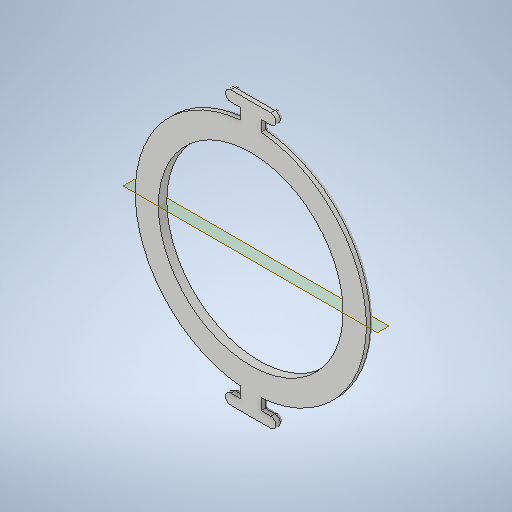
# Autodesk Inventor part: Baseplate_mitte
Saved by Autodesk Inventor 2025 (Build 290162000, 162)
## iProperties
Created: 2020-01-15
Part Number: Baseplate_mitte
Material: Generisch
Document SubType Name: Modeling
Designer: maxse
Density: 1 g/cm^3
Appearance: Vorgabe
Author: maxse
Autodesk Inventor part; units mm, degrees
(part 1 of 2)
ref_plane "YZ Plane" through (0, 0, 0) normal (1, 0, 0) x (0, 1, 0)
ref_plane "XZ Plane" through (0, 0, 0) normal (0, 1, 0) x (-1, 0, 0)
ref_plane "XY Plane" through (0, 0, 0) normal (0, 0, 1) x (1, 0, 0)
sketch "Skizze1" plane through (0, 0, 0) normal (0, 1, 0) x (-1, 0, 0)
  circle A0 centre (0, 0) radius 55
  circle A1 centre (0, 0) radius 43.96
  line L0 (-9.5, -65) -> (9.5, -65)
  line L1 (-9.5, -60) -> (-5, -60)
  line L2 (-5, -60) -> (-5, -54.7723)
  line L3 (5, -54.7723) -> (5, -60)
  line L4 (5, -60) -> (9.5, -60)
  arc A2 (9.5, -65) -> (9.5, -60) centre (9.5, -62.5) ccw
  arc A3 (-9.5, -60) -> (-9.5, -65) centre (-9.5, -62.5) ccw
  dimension "d0" = 110
  dimension "d1" = 87.92
  dimension "d2" = 10
  dimension "d3" = 2.5
  dimension "d4" = 2.5
  dimension "d5" = 5
  dimension "d6" = 5
  dimension "d7" = 24
  dimension "d8" = 60
  dimension "d9" = 4.5
  constraints: 10 end point, 6 point on circle, 4 centre point, 2 coincident, 2 horizontal, 2 point on line, 1 parallel, 1 perpendicular
  measures "d0" diameter of A0
  measures "d1" diameter of A1
  measures "d2" distance between parallel lines of L3 L2
  measures "d3" radius of A2
  measures "d4" radius of A3
  measures "d5" distance between parallel lines of L1 L0
  measures "d6" distance from line of point (0, 0) L2
  measures "d8" distance from line of A0.centre L4
  measures "d9" distance from line of L3 A2.centre
extrude "Extrusion1" add sketch "Skizze1" along normal blind 4
mirror "Spiegeln1" about plane through (0, 0, 0) normal (0, 0, 1) of "Extrusion1"
fillet "Rundung2" radius 2 16 edges at (-55, 4, 0) (55, 4, 0) (5, 4, 57.3861) (-5, 4, 57.3861) (-12, 4, 62.5) (-7.25, 4, 60) (12, 4, 62.5) (7.25, 4, 60) (0, 4, 65) (-12, 4, -62.5) (-7.25, 4, -60) (12, 4, -62.5) (7.25, 4, -60) (0, 4, -65) (-5, 4, -57.3861) (5, 4, -57.3861)
sketch "Skizze2" plane through (0, 4, 0) normal (0, 1, 0) x (1, 0, 0)
  circle A0 centre (0, 0) radius 45 projected
  line L0 (-69.5668, 0) -> (60.0552, 0)
  spline S0 degree 2 poles (24.3984, -40.0383) (24.7167, -39.8443) (25.3552, -39.7162) (25.6461, -39.781) knots 0 0 0 1 2 2 2
  spline S1 degree 2 poles (25.6461, -39.781) (25.9314, -39.8443) (26.405, -40.201) (26.5674, -40.4675) knots 0 0 0 1 2 2 2
  spline S2 degree 2 poles (26.5674, -40.4675) (26.7782, -40.8135) (26.7622, -41.6204) (26.5147, -42.0084) knots 0 0 0 1 2 2 2
  line L1 (26.5147, -42.0084) -> (26.5253, -42.0257)
  spline S3 degree 2 poles (26.5253, -42.0257) (26.9519, -42.0172) (27.522, -42.2677) (27.7202, -42.5929) knots 0 0 0 1 2 2 2
  spline S4 degree 2 poles (27.7202, -42.5929) (28.0133, -43.0738) (27.6789, -44.1602) (27.1183, -44.5018) knots 0 0 0 1 2 2 2
  spline S5 degree 2 poles (27.1183, -44.5018) (26.5371, -44.856) (25.4636, -44.675) (25.1726, -44.1976) knots 0 0 0 1 2 2 2
  spline S6 degree 2 poles (25.1726, -44.1976) (24.9976, -43.9104) (24.9917, -43.1453) (25.2095, -42.7943) knots 0 0 0 1 2 2 2
  line L2 (25.2095, -42.7943) -> (25.199, -42.777)
  spline S7 degree 2 poles (25.199, -42.777) (24.7199, -42.8317) (24.0322, -42.5675) (23.7918, -42.173) knots 0 0 0 1 2 2 2
  spline S8 degree 2 poles (23.7918, -42.173) (23.4587, -41.6264) (23.8033, -40.401) (24.3984, -40.0383) knots 0 0 0 1 2 2 2
  spline S9 degree 2 poles (24.3463, -41.7592) (24.5065, -42.0222) (24.9039, -42.2071) (25.295, -42.187) knots 0 0 0 1 2 2 2
  spline S10 degree 2 poles (25.295, -42.187) (25.4256, -42.1834) (25.8289, -42.1132) (26.0836, -42.0718) knots 0 0 0 1 2 2 2
  spline S11 degree 2 poles (26.0836, -42.0718) (26.224, -41.7728) (26.1941, -41.1552) (26.0149, -40.8611) knots 0 0 0 1 2 2 2
  spline S12 degree 2 poles (26.0149, -40.8611) (25.7787, -40.4736) (25.0038, -40.253) (24.6508, -40.4681) knots 0 0 0 1 2 2 2
  spline S13 degree 2 poles (24.6508, -40.4681) (24.291, -40.6874) (24.1186, -41.3856) (24.3463, -41.7592) knots 0 0 0 1 2 2 2
  spline S14 degree 2 poles (25.7289, -43.8491) (25.9039, -44.1362) (26.522, -44.2863) (26.8646, -44.0775) knots 0 0 0 1 2 2 2
  spline S15 degree 2 poles (26.8646, -44.0775) (27.176, -43.8878) (27.3651, -43.3028) (27.1859, -43.0086) knots 0 0 0 1 2 2 2
  spline S16 degree 2 poles (27.1859, -43.0086) (27.0573, -42.7976) (26.6739, -42.6279) (26.3981, -42.6346) knots 0 0 0 1 2 2 2
  spline S17 degree 2 poles (26.3981, -42.6346) (26.2821, -42.6389) (25.812, -42.6929) (25.6337, -42.7351) knots 0 0 0 1 2 2 2
  spline S18 degree 2 poles (25.6337, -42.7351) (25.5006, -43.0772) (25.5708, -43.5896) (25.7289, -43.8491) knots 0 0 0 1 2 2 2
  line L3 (21.6421, -46.4852) -> (21.6582, -41.7158)
  line L4 (21.6582, -41.7158) -> (22.2948, -41.3944)
  line L5 (22.2948, -41.3944) -> (22.2433, -46.3633)
  line L6 (22.2433, -46.3633) -> (24.5473, -45.2002)
  line L7 (24.5473, -45.2002) -> (24.8121, -45.7246)
  line L8 (24.8121, -45.7246) -> (21.9799, -47.1544)
  line L9 (21.9799, -47.1544) -> (21.6421, -46.4852)
  line L10 (18.1735, -43.3461) -> (18.9107, -43.0296)
  line L11 (18.9107, -43.0296) -> (19.2879, -43.9083)
  line L12 (19.2879, -43.9083) -> (18.5507, -44.2248)
  line L13 (18.5507, -44.2248) -> (18.1735, -43.3461)
  spline S19 degree 2 poles (14.9287, -46.263) (14.8073, -45.9235) (14.8174, -45.2658) (14.9394, -44.9812) knots 0 0 0 1 2 2 2
  spline S20 degree 2 poles (14.9394, -44.9812) (15.0614, -44.6966) (15.5641, -44.2371) (15.9304, -44.1062) knots 0 0 0 1 2 2 2
  spline S21 degree 2 poles (15.9304, -44.1062) (16.2661, -43.9861) (16.9756, -43.9003) (17.2582, -43.9326) knots 0 0 0 1 2 2 2
  line L14 (17.2582, -43.9326) -> (17.497, -44.6003)
  line L15 (17.497, -44.6003) -> (17.4512, -44.6166)
  spline S22 degree 2 poles (17.4512, -44.6166) (17.3596, -44.5891) (17.0396, -44.5487) (16.8537, -44.5463) knots 0 0 0 1 2 2 2
  spline S23 degree 2 poles (16.8537, -44.5463) (16.6436, -44.5483) (16.3086, -44.5863) (16.114, -44.6558) knots 0 0 0 1 2 2 2
  spline S24 degree 2 poles (16.114, -44.6558) (15.9233, -44.7241) (15.6137, -44.9896) (15.5372, -45.1848) knots 0 0 0 1 2 2 2
  spline S25 degree 2 poles (15.5372, -45.1848) (15.4694, -45.3683) (15.481, -45.7858) (15.5711, -46.0376) knots 0 0 0 1 2 2 2
  spline S26 degree 2 poles (15.5711, -46.0376) (15.6611, -46.2895) (15.9131, -46.5608) (16.081, -46.6213) knots 0 0 0 1 2 2 2
  spline S27 degree 2 poles (16.081, -46.6213) (16.2568, -46.6918) (16.6891, -46.6491) (16.9294, -46.5632) knots 0 0 0 1 2 2 2
  spline S28 degree 2 poles (16.9294, -46.5632) (17.1889, -46.4704) (17.6753, -46.2061) (17.8194, -46.1158) knots 0 0 0 1 2 2 2
  line L16 (17.8194, -46.1158) -> (18.6871, -48.5424)
  line L17 (18.6871, -48.5424) -> (16.1041, -49.466)
  line L18 (16.1041, -49.466) -> (15.9063, -48.9127)
  line L19 (15.9063, -48.9127) -> (17.8826, -48.2061)
  line L20 (17.8826, -48.2061) -> (17.4338, -46.9508)
  spline S29 degree 2 poles (17.4338, -46.9508) (17.3248, -47.007) (17.1076, -47.0976) (17.016, -47.1303) knots 0 0 0 1 2 2 2
  spline S30 degree 2 poles (17.016, -47.1303) (16.6536, -47.2599) (16.1115, -47.3204) (15.8198, -47.2267) knots 0 0 0 1 2 2 2
  spline S31 degree 2 poles (15.8198, -47.2267) (15.5243, -47.1344) (15.0815, -46.6903) (14.9287, -46.263) knots 0 0 0 1 2 2 2
  line L21 (9.4987, -46.0663) -> (10.0195, -48.1748)
  spline S32 degree 2 poles (10.0195, -48.1748) (10.0817, -48.4265) (10.2269, -48.8456) (10.319, -48.948) knots 0 0 0 1 2 2 2
  spline S33 degree 2 poles (10.319, -48.948) (10.414, -49.0623) (10.685, -49.1289) (10.8935, -49.0774) knots 0 0 0 1 2 2 2
  spline S34 degree 2 poles (10.8935, -49.0774) (11.0823, -49.0308) (11.4577, -48.6918) (11.6315, -48.4152) knots 0 0 0 1 2 2 2
  spline S35 degree 2 poles (11.6315, -48.4152) (11.6139, -48.3611) (11.5682, -48.2096) (11.5429, -48.1073) knots 0 0 0 1 2 2 2
  line L22 (11.5429, -48.1073) -> (10.9502, -45.7078)
  line L23 (10.9502, -45.7078) -> (11.5638, -45.5562)
  line L24 (11.5638, -45.5562) -> (12.0846, -47.6646)
  spline S36 degree 2 poles (12.0846, -47.6646) (12.1468, -47.9164) (12.2921, -48.3354) (12.3842, -48.4379) knots 0 0 0 1 2 2 2
  spline S37 degree 2 poles (12.3842, -48.4379) (12.4792, -48.5522) (12.7502, -48.6188) (12.9587, -48.5673) knots 0 0 0 1 2 2 2
  spline S38 degree 2 poles (12.9587, -48.5673) (13.1554, -48.5187) (13.5308, -48.163) (13.6877, -47.9198) knots 0 0 0 1 2 2 2
  line L25 (13.6877, -47.9198) -> (13.0153, -45.1977)
  line L26 (13.0153, -45.1977) -> (13.629, -45.0461)
  line L27 (13.629, -45.0461) -> (14.5287, -48.6886)
  line L28 (14.5287, -48.6886) -> (13.9151, -48.8402)
  line L29 (13.9151, -48.8402) -> (13.816, -48.439)
  spline S39 degree 2 poles (13.816, -48.439) (13.6353, -48.7382) (13.2284, -49.1184) (12.9451, -49.1883) knots 0 0 0 1 2 2 2
  spline S40 degree 2 poles (12.9451, -49.1883) (12.6226, -49.268) (12.0501, -49.0964) (11.8377, -48.7941) knots 0 0 0 1 2 2 2
  spline S41 degree 2 poles (11.8377, -48.7941) (11.6352, -49.1738) (11.1868, -49.6227) (10.88, -49.6984) knots 0 0 0 1 2 2 2
  spline S42 degree 2 poles (10.88, -49.6984) (10.644, -49.7567) (10.2225, -49.7064) (10.0401, -49.5762) knots 0 0 0 1 2 2 2
  spline S43 degree 2 poles (10.0401, -49.5762) (9.8537, -49.4469) (9.57, -48.9911) (9.4777, -48.6174) knots 0 0 0 1 2 2 2
  line L30 (9.4777, -48.6174) -> (8.885, -46.2179)
  line L31 (8.885, -46.2179) -> (9.4987, -46.0663)
  line L32 (3.7893, -46.8825) -> (4.0482, -49.0389)
  spline S44 degree 2 poles (4.0482, -49.0389) (4.0791, -49.2963) (4.172, -49.73) (4.2508, -49.843) knots 0 0 0 1 2 2 2
  spline S45 degree 2 poles (4.2508, -49.843) (4.3311, -49.968) (4.592, -50.0673) (4.8052, -50.0417) knots 0 0 0 1 2 2 2
  spline S46 degree 2 poles (4.8052, -50.0417) (4.9983, -50.0185) (5.4123, -49.728) (5.6186, -49.4747) knots 0 0 0 1 2 2 2
  spline S47 degree 2 poles (5.6186, -49.4747) (5.6078, -49.4189) (5.5809, -49.263) (5.5684, -49.1584) knots 0 0 0 1 2 2 2
  line L33 (5.5684, -49.1584) -> (5.2738, -46.7043)
  line L34 (5.2738, -46.7043) -> (5.9014, -46.629)
  line L35 (5.9014, -46.629) -> (6.1602, -48.7853)
  spline S48 degree 2 poles (6.1602, -48.7853) (6.1911, -49.0428) (6.284, -49.4765) (6.3629, -49.5894) knots 0 0 0 1 2 2 2
  spline S49 degree 2 poles (6.3629, -49.5894) (6.4432, -49.7145) (6.704, -49.8137) (6.9172, -49.7882) knots 0 0 0 1 2 2 2
  spline S50 degree 2 poles (6.9172, -49.7882) (7.1184, -49.764) (7.5345, -49.457) (7.7201, -49.2347) knots 0 0 0 1 2 2 2
  line L36 (7.7201, -49.2347) -> (7.3859, -46.4508)
  line L37 (7.3859, -46.4508) -> (8.0135, -46.3755)
  line L38 (8.0135, -46.3755) -> (8.4606, -50.1008)
  line L39 (8.4606, -50.1008) -> (7.8331, -50.1761)
  line L40 (7.8331, -50.1761) -> (7.7838, -49.7658)
  spline S51 degree 2 poles (7.7838, -49.7658) (7.5679, -50.0406) (7.1175, -50.3681) (6.8278, -50.4029) knots 0 0 0 1 2 2 2
  spline S52 degree 2 poles (6.8278, -50.4029) (6.4979, -50.4425) (5.9508, -50.2021) (5.777, -49.8761) knots 0 0 0 1 2 2 2
  spline S53 degree 2 poles (5.777, -49.8761) (5.5295, -50.2282) (5.0295, -50.6187) (4.7157, -50.6564) knots 0 0 0 1 2 2 2
  spline S54 degree 2 poles (4.7157, -50.6564) (4.4744, -50.6854) (4.0622, -50.5839) (3.8971, -50.4323) knots 0 0 0 1 2 2 2
  spline S55 degree 2 poles (3.8971, -50.4323) (3.728, -50.2812) (3.5022, -49.7941) (3.4563, -49.4119) knots 0 0 0 1 2 2 2
  line L41 (3.4563, -49.4119) -> (3.1617, -46.9579)
  line L42 (3.1617, -46.9579) -> (3.7893, -46.8825)
  spline S56 degree 2 poles (-3.071, -48.9106) (-3.0447, -47.9709) (-2.1185, -46.8862) (-1.434, -46.9053) knots 0 0 0 1 2 2 2
  spline S57 degree 2 poles (-1.434, -46.9053) (-1.1545, -46.9131) (-0.7288, -47.0547) (-0.5098, -47.1946) knots 0 0 0 1 2 2 2
  line L43 (-0.5098, -47.1946) -> (-0.4658, -45.6231)
  line L44 (-0.4658, -45.6231) -> (0.166, -45.6408)
  line L45 (0.166, -45.6408) -> (0.0224, -50.7725)
  line L46 (0.0224, -50.7725) -> (-0.6094, -50.7548)
  line L47 (-0.6094, -50.7548) -> (-0.5984, -50.362)
  spline S58 degree 2 poles (-0.5984, -50.362) (-0.8393, -50.5701) (-1.4224, -50.8375) (-1.7586, -50.8281) knots 0 0 0 1 2 2 2
  spline S59 degree 2 poles (-1.7586, -50.8281) (-2.4026, -50.8101) (-3.095, -49.7692) (-3.071, -48.9106) knots 0 0 0 1 2 2 2
  spline S60 degree 2 poles (-2.4168, -48.8559) (-2.4348, -49.4999) (-2.0456, -50.2201) (-1.5879, -50.2329) knots 0 0 0 1 2 2 2
  spline S61 degree 2 poles (-1.5879, -50.2329) (-1.3206, -50.2404) (-0.8117, -50.0155) (-0.5837, -49.8354) knots 0 0 0 1 2 2 2
  line L48 (-0.5837, -49.8354) -> (-0.5241, -47.705)
  spline S62 degree 2 poles (-0.5241, -47.705) (-0.7679, -47.5806) (-1.1177, -47.4816) (-1.3446, -47.4753) knots 0 0 0 1 2 2 2
  spline S63 degree 2 poles (-1.3446, -47.4753) (-1.8346, -47.4616) (-2.3976, -48.1673) (-2.4168, -48.8559) knots 0 0 0 1 2 2 2
  spline S64 degree 2 poles (-5.2796, -46.6177) (-4.3852, -46.7137) (-3.5098, -47.8223) (-3.6092, -48.7489) knots 0 0 0 1 2 2 2
  spline S65 degree 2 poles (-3.6092, -48.7489) (-3.7069, -49.6594) (-4.7775, -50.6367) (-5.547, -50.5541) knots 0 0 0 1 2 2 2
  spline S66 degree 2 poles (-5.547, -50.5541) (-5.8935, -50.517) (-6.4077, -50.258) (-6.5822, -50.0233) knots 0 0 0 1 2 2 2
  spline S67 degree 2 poles (-6.5822, -50.0233) (-6.7607, -49.7882) (-6.9081, -49.1489) (-6.8601, -48.7017) knots 0 0 0 1 2 2 2
  line L49 (-6.8601, -48.7017) -> (-6.8234, -48.3593)
  line L50 (-6.8234, -48.3593) -> (-4.241, -48.6363)
  spline S68 degree 2 poles (-4.241, -48.6363) (-4.1714, -47.9876) (-4.7502, -47.2287) (-5.3303, -47.1665) knots 0 0 0 1 2 2 2
  spline S69 degree 2 poles (-5.3303, -47.1665) (-5.5358, -47.1445) (-5.9446, -47.1943) (-6.1135, -47.2496) knots 0 0 0 1 2 2 2
  spline S70 degree 2 poles (-6.1135, -47.2496) (-6.2913, -47.312) (-6.5401, -47.4279) (-6.6236, -47.4842) knots 0 0 0 1 2 2 2
  line L51 (-6.6236, -47.4842) -> (-6.6599, -47.4803)
  line L52 (-6.6599, -47.4803) -> (-6.5864, -46.7954)
  spline S71 degree 2 poles (-6.5864, -46.7954) (-6.4729, -46.7628) (-6.1287, -46.6693) (-5.9959, -46.6468) knots 0 0 0 1 2 2 2
  spline S72 degree 2 poles (-5.9959, -46.6468) (-5.809, -46.6139) (-5.5052, -46.5935) (-5.2796, -46.6177) knots 0 0 0 1 2 2 2
  spline S73 degree 2 poles (-6.2625, -48.9044) (-6.2816, -49.1591) (-6.2166, -49.5409) (-6.1293, -49.6766) knots 0 0 0 1 2 2 2
  spline S74 degree 2 poles (-6.1293, -49.6766) (-6.0357, -49.8293) (-5.7092, -50.0151) (-5.4554, -50.0423) knots 0 0 0 1 2 2 2
  spline S75 degree 2 poles (-5.4554, -50.0423) (-5.2056, -50.0691) (-4.8391, -49.9577) (-4.6785, -49.8282) knots 0 0 0 1 2 2 2
  spline S76 degree 2 poles (-4.6785, -49.8282) (-4.5215, -49.6942) (-4.3381, -49.3512) (-4.2924, -49.1157) knots 0 0 0 1 2 2 2
  line L53 (-4.2924, -49.1157) -> (-6.2625, -48.9044)
  spline S77 degree 2 poles (-8.3657, -46.1775) (-7.8585, -46.2644) (-7.3867, -46.9414) (-7.4942, -47.5684) knots 0 0 0 1 2 2 2
  line L54 (-7.4942, -47.5684) -> (-7.8455, -49.6171)
  line L55 (-7.8455, -49.6171) -> (-7.4262, -49.689)
  line L56 (-7.4262, -49.689) -> (-7.5145, -50.2042)
  line L57 (-7.5145, -50.2042) -> (-7.9338, -50.1323)
  line L58 (-7.9338, -50.1323) -> (-8.116, -51.1946)
  line L59 (-8.116, -51.1946) -> (-8.739, -51.0878)
  line L60 (-8.739, -51.0878) -> (-8.5568, -50.0255)
  line L61 (-8.5568, -50.0255) -> (-9.703, -49.829)
  line L62 (-9.703, -49.829) -> (-9.6146, -49.3138)
  line L63 (-9.6146, -49.3138) -> (-8.4685, -49.5103)
  line L64 (-8.4685, -49.5103) -> (-8.1665, -47.7491)
  spline S78 degree 2 poles (-8.1665, -47.7491) (-8.1186, -47.4696) (-8.0858, -47.1587) (-8.1311, -47.0152) knots 0 0 0 1 2 2 2
  spline S79 degree 2 poles (-8.1311, -47.0152) (-8.1672, -46.8898) (-8.3989, -46.7309) (-8.6146, -46.6939) knots 0 0 0 1 2 2 2
  spline S80 degree 2 poles (-8.6146, -46.6939) (-8.7663, -46.6679) (-9.0656, -46.7111) (-9.1343, -46.7281) knots 0 0 0 1 2 2 2
  line L65 (-9.1343, -46.7281) -> (-9.1703, -46.722)
  line L66 (-9.1703, -46.722) -> (-9.0744, -46.1629)
  spline S81 degree 2 poles (-9.0744, -46.1629) (-8.8905, -46.1451) (-8.5214, -46.1508) (-8.3657, -46.1775) knots 0 0 0 1 2 2 2
  line L67 (-12.1384, -48.5969) -> (-12.1068, -48.604)
  spline S82 degree 2 poles (-12.1068, -48.604) (-12.0401, -48.6397) (-11.8877, -48.6822) (-11.7809, -48.7062) knots 0 0 0 1 2 2 2
  spline S83 degree 2 poles (-11.7809, -48.7062) (-11.5318, -48.762) (-10.9928, -48.6546) (-10.7235, -48.4907) knots 0 0 0 1 2 2 2
  line L68 (-10.7235, -48.4907) -> (-10.1409, -45.8932)
  line L69 (-10.1409, -45.8932) -> (-9.5241, -46.0315)
  line L70 (-9.5241, -46.0315) -> (-10.3453, -49.6926)
  line L71 (-10.3453, -49.6926) -> (-10.9621, -49.5542)
  line L72 (-10.9621, -49.5542) -> (-10.8397, -49.0086)
  spline S84 degree 2 poles (-10.8397, -49.0086) (-11.2432, -49.2337) (-11.8003, -49.3662) (-12.0375, -49.313) knots 0 0 0 1 2 2 2
  spline S85 degree 2 poles (-12.0375, -49.313) (-12.1324, -49.2917) (-12.2255, -49.2625) (-12.2821, -49.2374) knots 0 0 0 1 2 2 2
  line L73 (-12.2821, -49.2374) -> (-12.1384, -48.5969)
  line L74 (-12.5586, -45.2922) -> (-11.9483, -45.457)
  line L75 (-11.9483, -45.457) -> (-12.9265, -49.0793)
  line L76 (-12.9265, -49.0793) -> (-13.5367, -48.9145)
  line L77 (-13.5367, -48.9145) -> (-12.5586, -45.2922)
  line L78 (-13.7425, -49.5052) -> (-13.0501, -49.6922)
  line L79 (-13.0501, -49.6922) -> (-13.2212, -50.3259)
  line L80 (-13.2212, -50.3259) -> (-13.9136, -50.1389)
  line L81 (-13.9136, -50.1389) -> (-13.7425, -49.5052)
  line L82 (-18.1924, -43.3603) -> (-17.6023, -43.5869)
  line L83 (-17.6023, -43.5869) -> (-17.7388, -43.9424)
  spline S86 degree 2 poles (-17.7388, -43.9424) (-17.5591, -43.8812) (-17.3005, -43.8069) (-17.1396, -43.7949) knots 0 0 0 1 2 2 2
  spline S87 degree 2 poles (-17.1396, -43.7949) (-16.9916, -43.7823) (-16.6983, -43.8211) (-16.5205, -43.8893) knots 0 0 0 1 2 2 2
  spline S88 degree 2 poles (-16.5205, -43.8893) (-16.2331, -43.9997) (-15.8404, -44.4239) (-15.7587, -44.72) knots 0 0 0 1 2 2 2
  spline S89 degree 2 poles (-15.7587, -44.72) (-15.6771, -45.0161) (-15.7494, -45.7696) (-15.9193, -46.2122) knots 0 0 0 1 2 2 2
  spline S90 degree 2 poles (-15.9193, -46.2122) (-16.0965, -46.6737) (-16.5933, -47.2555) (-16.8986, -47.429) knots 0 0 0 1 2 2 2
  spline S91 degree 2 poles (-16.8986, -47.429) (-17.1787, -47.5819) (-17.8198, -47.6353) (-18.1186, -47.5205) knots 0 0 0 1 2 2 2
  spline S92 degree 2 poles (-18.1186, -47.5205) (-18.3797, -47.4203) (-18.7242, -47.1535) (-18.8934, -46.9497) knots 0 0 0 1 2 2 2
  line L84 (-18.8934, -46.9497) -> (-19.4743, -48.4627)
  line L85 (-19.4743, -48.4627) -> (-20.0644, -48.2362)
  line L86 (-20.0644, -48.2362) -> (-18.1924, -43.3603)
  line L87 (-17.9291, -44.438) -> (-18.706, -46.4617)
  spline S93 degree 2 poles (-18.706, -46.4617) (-18.5273, -46.6518) (-18.2098, -46.8649) (-18.0093, -46.9419) knots 0 0 0 1 2 2 2
  spline S94 degree 2 poles (-18.0093, -46.9419) (-17.5554, -47.1161) (-16.7796, -46.6328) (-16.5327, -45.9897) knots 0 0 0 1 2 2 2
  spline S95 degree 2 poles (-16.5327, -45.9897) (-16.2945, -45.3693) (-16.4366, -44.5639) (-16.8717, -44.3969) knots 0 0 0 1 2 2 2
  spline S96 degree 2 poles (-16.8717, -44.3969) (-17.1024, -44.3083) (-17.6528, -44.3401) (-17.9291, -44.438) knots 0 0 0 1 2 2 2
  line L88 (-19.6119, -42.7139) -> (-19.0357, -42.9737)
  line L89 (-19.0357, -42.9737) -> (-20.5783, -46.394)
  line L90 (-20.5783, -46.394) -> (-21.1545, -46.1341)
  line L91 (-21.1545, -46.1341) -> (-19.6119, -42.7139)
  line L92 (-21.4517, -46.6846) -> (-20.7979, -46.9794)
  line L93 (-20.7979, -46.9794) -> (-21.0678, -47.5778)
  line L94 (-21.0678, -47.5778) -> (-21.7216, -47.2829)
  line L95 (-21.7216, -47.2829) -> (-21.4517, -46.6846)
  spline S97 degree 2 poles (-21.3169, -41.7878) (-20.9815, -41.9595) (-20.4931, -42.4371) (-20.3536, -42.6359) knots 0 0 0 1 2 2 2
  line L96 (-20.3536, -42.6359) -> (-20.6766, -43.2671)
  line L97 (-20.6766, -43.2671) -> (-20.7055, -43.2523)
  spline S98 degree 2 poles (-20.7055, -43.2523) (-20.7481, -43.1577) (-20.8727, -42.921) (-20.9963, -42.7621) knots 0 0 0 1 2 2 2
  spline S99 degree 2 poles (-20.9963, -42.7621) (-21.1019, -42.6216) (-21.3964, -42.3434) (-21.5804, -42.2493) knots 0 0 0 1 2 2 2
  spline S100 degree 2 poles (-21.5804, -42.2493) (-21.7138, -42.1809) (-22.0518, -42.0854) (-22.1498, -42.0989) knots 0 0 0 1 2 2 2
  spline S101 degree 2 poles (-22.1498, -42.0989) (-22.2895, -42.1139) (-22.4626, -42.221) (-22.5438, -42.3797) knots 0 0 0 1 2 2 2
  spline S102 degree 2 poles (-22.5438, -42.3797) (-22.6454, -42.5781) (-22.5342, -42.8945) (-22.2915, -43.1051) knots 0 0 0 1 2 2 2
  spline S103 degree 2 poles (-22.2915, -43.1051) (-22.1962, -43.1858) (-21.8869, -43.4351) (-21.7593, -43.5505) knots 0 0 0 1 2 2 2
  spline S104 degree 2 poles (-21.7593, -43.5505) (-21.4342, -43.858) (-21.3243, -44.4969) (-21.4922, -44.8251) knots 0 0 0 1 2 2 2
  spline S105 degree 2 poles (-21.4922, -44.8251) (-21.7249, -45.2796) (-22.6964, -45.497) (-23.2591, -45.209) knots 0 0 0 1 2 2 2
  spline S106 degree 2 poles (-23.2591, -45.209) (-23.5368, -45.0668) (-24.0293, -44.6418) (-24.1669, -44.4393) knots 0 0 0 1 2 2 2
  line L98 (-24.1669, -44.4393) -> (-23.8587, -43.837)
  line L99 (-23.8587, -43.837) -> (-23.8298, -43.8518)
  spline S107 degree 2 poles (-23.8298, -43.8518) (-23.702, -44.1357) (-23.2769, -44.6036) (-23.0064, -44.742) knots 0 0 0 1 2 2 2
  spline S108 degree 2 poles (-23.0064, -44.742) (-22.7287, -44.8842) (-22.2264, -44.8454) (-22.1064, -44.6109) knots 0 0 0 1 2 2 2
  spline S109 degree 2 poles (-22.1064, -44.6109) (-21.9974, -44.3981) (-22.1195, -44.0762) (-22.3387, -43.8821) knots 0 0 0 1 2 2 2
  spline S110 degree 2 poles (-22.3387, -43.8821) (-22.4447, -43.7869) (-22.7217, -43.5632) (-22.8709, -43.4367) knots 0 0 0 1 2 2 2
  spline S111 degree 2 poles (-22.8709, -43.4367) (-23.1908, -43.1547) (-23.3463, -42.5335) (-23.1561, -42.1619) knots 0 0 0 1 2 2 2
  spline S112 degree 2 poles (-23.1561, -42.1619) (-23.0453, -41.9455) (-22.6801, -41.65) (-22.4422, -41.5942) knots 0 0 0 1 2 2 2
  spline S113 degree 2 poles (-22.4422, -41.5942) (-22.1898, -41.5368) (-21.6596, -41.6124) (-21.3169, -41.7878) knots 0 0 0 1 2 2 2
  line L100 (-25.6934, -39.3835) -> (-25.1534, -39.712)
  line L101 (-25.1534, -39.712) -> (-26.2651, -41.5398)
  spline S114 degree 2 poles (-26.2651, -41.5398) (-26.3998, -41.7614) (-26.5899, -42.1675) (-26.597, -42.3196) knots 0 0 0 1 2 2 2
  spline S115 degree 2 poles (-26.597, -42.3196) (-26.605, -42.4808) (-26.4411, -42.7416) (-26.2403, -42.8638) knots 0 0 0 1 2 2 2
  spline S116 degree 2 poles (-26.2403, -42.8638) (-26.0396, -42.9859) (-25.4832, -43.0302) (-25.1737, -42.9814) knots 0 0 0 1 2 2 2
  line L102 (-25.1737, -42.9814) -> (-23.7167, -40.5857)
  line L103 (-23.7167, -40.5857) -> (-23.1766, -40.9142)
  line L104 (-23.1766, -40.9142) -> (-25.8906, -45.3765)
  line L105 (-25.8906, -45.3765) -> (-26.4307, -45.0481)
  line L106 (-26.4307, -45.0481) -> (-25.4495, -43.4349)
  spline S117 degree 2 poles (-25.4495, -43.4349) (-25.8245, -43.5056) (-26.4308, -43.4498) (-26.6939, -43.2898) knots 0 0 0 1 2 2 2
  spline S118 degree 2 poles (-26.6939, -43.2898) (-27.1647, -43.0034) (-27.3188, -42.0561) (-26.9588, -41.4641) knots 0 0 0 1 2 2 2
  line L107 (-26.9588, -41.4641) -> (-25.6934, -39.3835)
  point P0 (0, 0)
  constraints: 2 end point, 1 horizontal, 2 other
extrude "Extrusion2" add sketch "Skizze2" along normal blind 1 contours S0 S1 S2 L1 S3 S4 S5 S6 L2 S7 S8 | L3 L4 L5 L6 L7 L8 L9 | L10 L11 L12 L13 | S19 S20 S21 L14 L15 S22 S23 S24 S25 S26 S27 S28 L16 L17 L18 L19 L20 S29 S30 S31 | L21 S32 S33 S34 S35 L22 L23 L24 S36 S37 S38 L25 L26 L27 L28 L29 S39 S40 S41 S42 S43 L30 L31 | L32 S44 S45 S46 S47 L33 L34 L35 S48 S49 S50 L36 L37 L38 L39 L40 S51 S52 S53 S54 S55 L41 L42 | S56 S57 L43 L44 L45 L46 L47 S58 S59 | S64 S65 S66 S67 L49 L50 S68 S69 S70 L51 L52 S71 S72 | S77 L54 L55 L56 L57 L58 L59 L60 L61 L62 L63 L64 S78 S79 S80 L65 L66 S81 | L67 S82 S83 L68 L69 L70 L71 L72 S84 S85 L73 | L74 L75 L76 L77 | L78 L79 L80 L81 | L82 L83 S86 S87 S88 S89 S90 S91 S92 L84 L85 L86 | L88 L89 L90 L91 | L92 L93 L94 L95 | S97 L96 L97 S98 S99 S100 S101 S102 S103 S104 S105 S106 L98 L99 S107 S108 S109 S110 S111 S112 S113 | L100 L101 S114 S115 S116 L102 L103 L104 L105 L106 S117 S118 L107
sketch "Skizze3" plane through (0, 4, 0) normal (0, 1, 0) x (1, 0, 0)
  circle A0 centre (0, 0) radius 45.2717
  spline S0 degree 2 poles (28.1118, 38.7127) (28.2498, 38.8928) (28.6266, 39.1186) (28.8277, 39.1431) knots 0 0 0 1 2 2 2
  spline S1 degree 2 poles (28.8277, 39.1431) (29.0804, 39.1745) (29.582, 39.0223) (29.8792, 38.7946) knots 0 0 0 1 2 2 2
  line L0 (29.8792, 38.7946) -> (30.1921, 38.5547)
  line L1 (30.1921, 38.5547) -> (30.9858, 39.5902)
  line L2 (30.9858, 39.5902) -> (31.355, 39.3072)
  line L3 (31.355, 39.3072) -> (29.2257, 36.5294)
  line L4 (29.2257, 36.5294) -> (28.5279, 37.0643)
  spline S2 degree 2 poles (28.5279, 37.0643) (28.2803, 37.2541) (27.9957, 37.6009) (27.9337, 37.795) knots 0 0 0 1 2 2 2
  spline S3 degree 2 poles (27.9337, 37.795) (27.8594, 38.0198) (27.934, 38.4808) (28.1118, 38.7127) knots 0 0 0 1 2 2 2
  spline S4 degree 2 poles (28.5053, 38.4289) (28.3949, 38.2848) (28.3318, 37.9973) (28.3813, 37.8521) knots 0 0 0 1 2 2 2
  spline S5 degree 2 poles (28.3813, 37.8521) (28.4242, 37.7263) (28.6221, 37.4996) (28.7954, 37.3667) knots 0 0 0 1 2 2 2
  line L5 (28.7954, 37.3667) -> (29.1016, 37.132)
  line L6 (29.1016, 37.132) -> (29.9505, 38.2396)
  line L7 (29.9505, 38.2396) -> (29.6984, 38.4328)
  spline S6 degree 2 poles (29.6984, 38.4328) (29.4733, 38.6054) (29.1412, 38.7456) (28.9787, 38.72) knots 0 0 0 1 2 2 2
  spline S7 degree 2 poles (28.9787, 38.72) (28.8315, 38.7006) (28.6071, 38.5617) (28.5053, 38.4289) knots 0 0 0 1 2 2 2
  spline S8 degree 2 poles (27.9009, 41.4872) (27.9678, 41.4894) (28.1977, 41.5034) (28.292, 41.4902) knots 0 0 0 1 2 2 2
  spline S9 degree 2 poles (28.292, 41.4902) (28.4231, 41.4757) (28.64, 41.4057) (28.8036, 41.2932) knots 0 0 0 1 2 2 2
  spline S10 degree 2 poles (28.8036, 41.2932) (28.9368, 41.2016) (29.1084, 40.9356) (29.1369, 40.7817) knots 0 0 0 1 2 2 2
  spline S11 degree 2 poles (29.1369, 40.7817) (29.1623, 40.6335) (29.0874, 40.2994) (28.9878, 40.1545) knots 0 0 0 1 2 2 2
  spline S12 degree 2 poles (28.9878, 40.1545) (28.8335, 39.9302) (28.4256, 39.7425) (28.1573, 39.7928) knots 0 0 0 1 2 2 2
  spline S13 degree 2 poles (28.1573, 39.7928) (27.9171, 39.834) (27.3783, 40.1117) (27.0796, 40.293) knots 0 0 0 1 2 2 2
  line L8 (27.0796, 40.293) -> (27.0314, 40.2229)
  spline S14 degree 2 poles (27.0314, 40.2229) (26.9446, 40.0967) (26.914, 39.8871) (26.9536, 39.7945) knots 0 0 0 1 2 2 2
  spline S15 degree 2 poles (26.9536, 39.7945) (26.9932, 39.7018) (27.1749, 39.5356) (27.2824, 39.4616) knots 0 0 0 1 2 2 2
  spline S16 degree 2 poles (27.2824, 39.4616) (27.4086, 39.3749) (27.8012, 39.215) (28.0216, 39.1701) knots 0 0 0 1 2 2 2
  line L9 (28.0216, 39.1701) -> (28.0427, 39.1556)
  line L10 (28.0427, 39.1556) -> (27.7871, 38.7841)
  spline S17 degree 2 poles (27.7871, 38.7841) (27.6673, 38.8251) (27.2429, 39.0138) (27.0582, 39.1408) knots 0 0 0 1 2 2 2
  spline S18 degree 2 poles (27.0582, 39.1408) (26.8339, 39.295) (26.576, 39.5757) (26.5171, 39.7504) knots 0 0 0 1 2 2 2
  spline S19 degree 2 poles (26.5171, 39.7504) (26.459, 39.9212) (26.5366, 40.2843) (26.6765, 40.4876) knots 0 0 0 1 2 2 2
  line L11 (26.6765, 40.4876) -> (27.6939, 41.9669)
  line L12 (27.6939, 41.9669) -> (28.0584, 41.7162)
  line L13 (28.0584, 41.7162) -> (27.9009, 41.4872)
  line L14 (27.692, 41.1834) -> (27.2789, 40.5828)
  spline S20 degree 2 poles (27.2789, 40.5828) (27.4178, 40.5045) (27.8401, 40.2726) (27.9897, 40.2248) knots 0 0 0 1 2 2 2
  spline S21 degree 2 poles (27.9897, 40.2248) (28.1651, 40.1695) (28.4814, 40.224) (28.5939, 40.3876) knots 0 0 0 1 2 2 2
  spline S22 degree 2 poles (28.5939, 40.3876) (28.7224, 40.5745) (28.6423, 40.9085) (28.4413, 41.0467) knots 0 0 0 1 2 2 2
  spline S23 degree 2 poles (28.4413, 41.0467) (28.2707, 41.164) (27.889, 41.2097) (27.692, 41.1834) knots 0 0 0 1 2 2 2
  line L15 (24.8465, 41.2165) -> (24.8658, 41.2044)
  spline S24 degree 2 poles (24.8658, 41.2044) (24.9015, 41.1653) (24.9922, 41.1017) (25.0571, 41.0611) knots 0 0 0 1 2 2 2
  spline S25 degree 2 poles (25.0571, 41.0611) (25.2084, 40.9661) (25.5893, 40.9115) (25.8052, 40.9568) knots 0 0 0 1 2 2 2
  line L16 (25.8052, 40.9568) -> (26.7952, 42.5356)
  line L17 (26.7952, 42.5356) -> (27.17, 42.3006)
  line L18 (27.17, 42.3006) -> (25.7748, 40.0754)
  line L19 (25.7748, 40.0754) -> (25.3999, 40.3104)
  line L20 (25.3999, 40.3104) -> (25.6078, 40.6421)
  spline S26 degree 2 poles (25.6078, 40.6421) (25.2891, 40.5875) (24.8905, 40.6299) (24.7463, 40.7203) knots 0 0 0 1 2 2 2
  spline S27 degree 2 poles (24.7463, 40.7203) (24.6886, 40.7564) (24.634, 40.7974) (24.6024, 40.8272) knots 0 0 0 1 2 2 2
  line L21 (24.6024, 40.8272) -> (24.8465, 41.2165)
  line L22 (25.3037, 43.4398) -> (25.6851, 43.2154)
  line L23 (25.6851, 43.2154) -> (24.3531, 40.9518)
  line L24 (24.3531, 40.9518) -> (23.9718, 41.1762)
  line L25 (23.9718, 41.1762) -> (25.3037, 43.4398)
  line L26 (23.7234, 40.8156) -> (24.156, 40.561)
  line L27 (24.156, 40.561) -> (23.923, 40.165)
  line L28 (23.923, 40.165) -> (23.4904, 40.4195)
  line L29 (23.4904, 40.4195) -> (23.7234, 40.8156)
  spline S28 degree 2 poles (24.1505, 44.162) (24.382, 44.0356) (24.7149, 43.6924) (24.8088, 43.5507) knots 0 0 0 1 2 2 2
  line L30 (24.8088, 43.5507) -> (24.5711, 43.115)
  line L31 (24.5711, 43.115) -> (24.5512, 43.1258)
  spline S29 degree 2 poles (24.5512, 43.1258) (24.5231, 43.1929) (24.4403, 43.3608) (24.3568, 43.4743) knots 0 0 0 1 2 2 2
  spline S30 degree 2 poles (24.3568, 43.4743) (24.2855, 43.5745) (24.0845, 43.7747) (23.9576, 43.844) knots 0 0 0 1 2 2 2
  spline S31 degree 2 poles (23.9576, 43.844) (23.8654, 43.8943) (23.6307, 43.9674) (23.5619, 43.9597) knots 0 0 0 1 2 2 2
  spline S32 degree 2 poles (23.5619, 43.9597) (23.4639, 43.9518) (23.3407, 43.8801) (23.2809, 43.7706) knots 0 0 0 1 2 2 2
  spline S33 degree 2 poles (23.2809, 43.7706) (23.2062, 43.6336) (23.2782, 43.4102) (23.444, 43.2583) knots 0 0 0 1 2 2 2
  spline S34 degree 2 poles (23.444, 43.2583) (23.5092, 43.2001) (23.7211, 43.0199) (23.8082, 42.9368) knots 0 0 0 1 2 2 2
  spline S35 degree 2 poles (23.8082, 42.9368) (24.03, 42.7156) (24.0951, 42.2664) (23.9714, 42.0399) knots 0 0 0 1 2 2 2
  spline S36 degree 2 poles (23.9714, 42.0399) (23.8002, 41.7262) (23.1164, 41.5921) (22.728, 41.804) knots 0 0 0 1 2 2 2
  spline S37 degree 2 poles (22.728, 41.804) (22.5363, 41.9087) (22.1995, 42.2152) (22.107, 42.3594) knots 0 0 0 1 2 2 2
  line L32 (22.107, 42.3594) -> (22.3339, 42.7752)
  line L33 (22.3339, 42.7752) -> (22.3538, 42.7644)
  spline S38 degree 2 poles (22.3538, 42.7644) (22.4379, 42.5633) (22.7267, 42.228) (22.9134, 42.1261) knots 0 0 0 1 2 2 2
  spline S39 degree 2 poles (22.9134, 42.1261) (23.1051, 42.0215) (23.4574, 42.0393) (23.5457, 42.2011) knots 0 0 0 1 2 2 2
  spline S40 degree 2 poles (23.5457, 42.2011) (23.6258, 42.348) (23.5464, 42.5755) (23.3966, 42.7155) knots 0 0 0 1 2 2 2
  spline S41 degree 2 poles (23.3966, 42.7155) (23.3242, 42.7841) (23.1345, 42.9457) (23.0325, 43.037) knots 0 0 0 1 2 2 2
  spline S42 degree 2 poles (23.0325, 43.037) (22.8138, 43.2403) (22.7166, 43.6779) (22.8565, 43.9343) knots 0 0 0 1 2 2 2
  spline S43 degree 2 poles (22.8565, 43.9343) (22.9381, 44.0837) (23.1991, 44.2837) (23.3666, 44.3183) knots 0 0 0 1 2 2 2
  spline S44 degree 2 poles (23.3666, 44.3183) (23.5443, 44.3538) (23.914, 44.2911) (24.1505, 44.162) knots 0 0 0 1 2 2 2
  line L34 (19.6249, 46.2981) -> (21.4728, 45.4629)
  line L35 (21.4728, 45.4629) -> (20.0313, 42.2735)
  line L36 (20.0313, 42.2735) -> (19.6074, 42.4651)
  line L37 (19.6074, 42.4651) -> (20.8784, 45.2771)
  line L38 (20.8784, 45.2771) -> (19.4543, 45.9208)
  line L39 (19.4543, 45.9208) -> (19.6249, 46.2981)
  spline S45 degree 2 poles (16.828, 45.9905) (17.0709, 46.6082) (17.9295, 47.0477) (18.4258, 46.8525) knots 0 0 0 1 2 2 2
  spline S46 degree 2 poles (18.4258, 46.8525) (18.9352, 46.6522) (19.2455, 45.7285) (19.0109, 45.132) knots 0 0 0 1 2 2 2
  spline S47 degree 2 poles (19.0109, 45.132) (18.77, 44.5197) (17.9014, 44.078) (17.4105, 44.2711) knots 0 0 0 1 2 2 2
  spline S48 degree 2 poles (17.4105, 44.2711) (16.9143, 44.4663) (16.5861, 45.3755) (16.828, 45.9905) knots 0 0 0 1 2 2 2
  spline S49 degree 2 poles (17.253, 45.8234) (17.0661, 45.3483) (17.2302, 44.7504) (17.5496, 44.6248) knots 0 0 0 1 2 2 2
  spline S50 degree 2 poles (17.5496, 44.6248) (17.869, 44.4992) (18.3991, 44.824) (18.5859, 45.2992) knots 0 0 0 1 2 2 2
  spline S51 degree 2 poles (18.5859, 45.2992) (18.7676, 45.7611) (18.606, 46.3732) (18.2867, 46.4988) knots 0 0 0 1 2 2 2
  spline S52 degree 2 poles (18.2867, 46.4988) (17.9699, 46.6234) (17.4378, 46.2932) (17.253, 45.8234) knots 0 0 0 1 2 2 2
  line L40 (14.9654, 48.0032) -> (15.385, 47.863)
  line L41 (15.385, 47.863) -> (15.3006, 47.6101)
  spline S53 degree 2 poles (15.3006, 47.6101) (15.4244, 47.6585) (15.6029, 47.7185) (15.715, 47.7319) knots 0 0 0 1 2 2 2
  spline S54 degree 2 poles (15.715, 47.7319) (15.8182, 47.7453) (16.0245, 47.7272) (16.1509, 47.685) knots 0 0 0 1 2 2 2
  spline S55 degree 2 poles (16.1509, 47.685) (16.3554, 47.6167) (16.6431, 47.3323) (16.7094, 47.1277) knots 0 0 0 1 2 2 2
  spline S56 degree 2 poles (16.7094, 47.1277) (16.7756, 46.9232) (16.7485, 46.394) (16.6433, 46.0793) knots 0 0 0 1 2 2 2
  spline S57 degree 2 poles (16.6433, 46.0793) (16.5337, 45.7511) (16.2043, 45.3288) (15.9962, 45.198) knots 0 0 0 1 2 2 2
  spline S58 degree 2 poles (15.9962, 45.198) (15.8051, 45.0824) (15.3584, 45.0252) (15.1459, 45.0962) knots 0 0 0 1 2 2 2
  spline S59 degree 2 poles (15.1459, 45.0962) (14.9602, 45.1582) (14.711, 45.3341) (14.5864, 45.4714) knots 0 0 0 1 2 2 2
  line L42 (14.5864, 45.4714) -> (14.227, 44.3953)
  line L43 (14.227, 44.3953) -> (13.8074, 44.5354)
  line L44 (13.8074, 44.5354) -> (14.9654, 48.0032)
  line L45 (15.1829, 47.2577) -> (14.7023, 45.8184)
  spline S60 degree 2 poles (14.7023, 45.8184) (14.8332, 45.691) (15.0618, 45.5518) (15.2044, 45.5042) knots 0 0 0 1 2 2 2
  spline S61 degree 2 poles (15.2044, 45.5042) (15.5272, 45.3964) (16.0548, 45.7585) (16.2075, 46.2158) knots 0 0 0 1 2 2 2
  spline S62 degree 2 poles (16.2075, 46.2158) (16.3548, 46.657) (16.2305, 47.2159) (15.9211, 47.3192) knots 0 0 0 1 2 2 2
  spline S63 degree 2 poles (15.9211, 47.3192) (15.757, 47.374) (15.3731, 47.3347) (15.1829, 47.2577) knots 0 0 0 1 2 2 2
  line L46 (12.4193, 46.4963) -> (12.4412, 46.4901)
  spline S64 degree 2 poles (12.4412, 46.4901) (12.4863, 46.4624) (12.5911, 46.4266) (12.6648, 46.4055) knots 0 0 0 1 2 2 2
  spline S65 degree 2 poles (12.6648, 46.4055) (12.8366, 46.3564) (13.2176, 46.4096) (13.4124, 46.5132) knots 0 0 0 1 2 2 2
  line L47 (13.4124, 46.5132) -> (13.9249, 48.3048)
  line L48 (13.9249, 48.3048) -> (14.3503, 48.1832)
  line L49 (14.3503, 48.1832) -> (13.628, 45.658)
  line L50 (13.628, 45.658) -> (13.2026, 45.7797)
  line L51 (13.2026, 45.7797) -> (13.3103, 46.156)
  spline S66 degree 2 poles (13.3103, 46.156) (13.0192, 46.015) (12.6245, 45.945) (12.4609, 45.9918) knots 0 0 0 1 2 2 2
  spline S67 degree 2 poles (12.4609, 45.9918) (12.3954, 46.0105) (12.3316, 46.0347) (12.293, 46.0546) knots 0 0 0 1 2 2 2
  line L52 (12.293, 46.0546) -> (12.4193, 46.4963)
  spline S68 degree 2 poles (10.2752, 47.8825) (10.4299, 48.5279) (11.2191, 49.0824) (11.7377, 48.9581) knots 0 0 0 1 2 2 2
  spline S69 degree 2 poles (11.7377, 48.9581) (12.27, 48.8304) (12.7056, 47.9589) (12.5561, 47.3356) knots 0 0 0 1 2 2 2
  spline S70 degree 2 poles (12.5561, 47.3356) (12.4027, 46.6957) (11.6039, 46.1376) (11.0909, 46.2606) knots 0 0 0 1 2 2 2
  spline S71 degree 2 poles (11.0909, 46.2606) (10.5723, 46.385) (10.1211, 47.2399) (10.2752, 47.8825) knots 0 0 0 1 2 2 2
  spline S72 degree 2 poles (10.7192, 47.776) (10.6002, 47.2796) (10.8457, 46.7103) (11.1795, 46.6302) knots 0 0 0 1 2 2 2
  spline S73 degree 2 poles (11.1795, 46.6302) (11.5132, 46.5502) (11.993, 46.9456) (12.1121, 47.442) knots 0 0 0 1 2 2 2
  spline S74 degree 2 poles (12.1121, 47.442) (12.2278, 47.9247) (11.9828, 48.5085) (11.649, 48.5885) knots 0 0 0 1 2 2 2
  spline S75 degree 2 poles (11.649, 48.5885) (11.3181, 48.6679) (10.8369, 48.267) (10.7192, 47.776) knots 0 0 0 1 2 2 2
  line L53 (8.1091, 49.6243) -> (8.5442, 49.5439)
  line L54 (8.5442, 49.5439) -> (8.2721, 48.0713)
  spline S76 degree 2 poles (8.2721, 48.0713) (8.2391, 47.8928) (8.2159, 47.5798) (8.2491, 47.4785) knots 0 0 0 1 2 2 2
  spline S77 degree 2 poles (8.2491, 47.4785) (8.2841, 47.3711) (8.4562, 47.2412) (8.618, 47.2113) knots 0 0 0 1 2 2 2
  spline S78 degree 2 poles (8.618, 47.2113) (8.7798, 47.1814) (9.1548, 47.291) (9.3451, 47.4) knots 0 0 0 1 2 2 2
  line L55 (9.3451, 47.4) -> (9.7016, 49.3301)
  line L56 (9.7016, 49.3301) -> (10.1367, 49.2497)
  line L57 (10.1367, 49.2497) -> (9.6596, 46.667)
  line L58 (9.6596, 46.667) -> (9.2245, 46.7474)
  line L59 (9.2245, 46.7474) -> (9.2776, 47.0347)
  spline S79 degree 2 poles (9.2776, 47.0347) (9.0499, 46.895) (8.6393, 46.7805) (8.4274, 46.8197) knots 0 0 0 1 2 2 2
  spline S80 degree 2 poles (8.4274, 46.8197) (8.0481, 46.8897) (7.7113, 47.4711) (7.7994, 47.9481) knots 0 0 0 1 2 2 2
  line L60 (7.7994, 47.9481) -> (8.1091, 49.6243)
  spline S81 degree 2 poles (4.7627, 50.1197) (5.0704, 50.0905) (5.5126, 49.8861) (5.6582, 49.7098) knots 0 0 0 1 2 2 2
  spline S82 degree 2 poles (5.6582, 49.7098) (5.8246, 49.5117) (5.926, 48.9892) (5.8905, 48.6165) knots 0 0 0 1 2 2 2
  line L61 (5.8905, 48.6165) -> (5.684, 46.4423)
  line L62 (5.684, 46.4423) -> (5.2209, 46.4863)
  line L63 (5.2209, 46.4863) -> (5.4275, 48.6605)
  spline S83 degree 2 poles (5.4275, 48.6605) (5.4505, 48.9033) (5.4195, 49.2368) (5.3446, 49.3778) knots 0 0 0 1 2 2 2
  spline S84 degree 2 poles (5.3446, 49.3778) (5.2649, 49.5278) (4.9566, 49.7024) (4.7251, 49.7244) knots 0 0 0 1 2 2 2
  spline S85 degree 2 poles (4.7251, 49.7244) (4.5077, 49.745) (4.1552, 49.6332) (4.0486, 49.5009) knots 0 0 0 1 2 2 2
  spline S86 degree 2 poles (4.0486, 49.5009) (3.9485, 49.3765) (3.8555, 49.0577) (3.8332, 48.8233) knots 0 0 0 1 2 2 2
  line L64 (3.8332, 48.8233) -> (3.6256, 46.6379)
  line L65 (3.6256, 46.6379) -> (3.1625, 46.6819)
  line L66 (3.1625, 46.6819) -> (3.3691, 48.856)
  spline S87 degree 2 poles (3.3691, 48.856) (3.4037, 49.2203) (3.5999, 49.7259) (3.8031, 49.8861) knots 0 0 0 1 2 2 2
  spline S88 degree 2 poles (3.8031, 49.8861) (3.9853, 50.034) (4.4408, 50.1503) (4.7627, 50.1197) knots 0 0 0 1 2 2 2
  line L67 (0.8016, 50.2761) -> (1.2438, 50.2599)
  line L68 (1.2438, 50.2599) -> (1.1889, 48.7633)
  spline S89 degree 2 poles (1.1889, 48.7633) (1.1823, 48.5819) (1.2048, 48.2689) (1.2524, 48.1735) knots 0 0 0 1 2 2 2
  spline S90 degree 2 poles (1.2524, 48.1735) (1.3027, 48.0723) (1.4919, 47.9689) (1.6563, 47.9629) knots 0 0 0 1 2 2 2
  spline S91 degree 2 poles (1.6563, 47.9629) (1.8206, 47.9568) (2.1757, 48.1198) (2.3481, 48.2554) knots 0 0 0 1 2 2 2
  line L69 (2.3481, 48.2554) -> (2.4201, 50.2168)
  line L70 (2.4201, 50.2168) -> (2.8622, 50.2006)
  line L71 (2.8622, 50.2006) -> (2.766, 47.5759)
  line L72 (2.766, 47.5759) -> (2.3238, 47.5921)
  line L73 (2.3238, 47.5921) -> (2.3345, 47.8841)
  spline S92 degree 2 poles (2.3345, 47.8841) (2.1296, 47.7128) (1.7401, 47.5397) (1.5247, 47.5476) knots 0 0 0 1 2 2 2
  spline S93 degree 2 poles (1.5247, 47.5476) (1.1392, 47.5618) (0.7214, 48.088) (0.7392, 48.5726) knots 0 0 0 1 2 2 2
  line L74 (0.7392, 48.5726) -> (0.8016, 50.2761)
  line L75 (-0.2705, 50.2715) -> (0.172, 50.2719)
  line L76 (0.172, 50.2719) -> (0.1746, 47.6455)
  line L77 (0.1746, 47.6455) -> (-0.2679, 47.6451)
  line L78 (-0.2679, 47.6451) -> (-0.2705, 50.2715)
  line L79 (-0.2987, 47.2083) -> (0.2034, 47.2087)
  line L80 (0.2034, 47.2087) -> (0.2038, 46.7493)
  line L81 (0.2038, 46.7493) -> (-0.2982, 46.7488)
  line L82 (-0.2982, 46.7488) -> (-0.2987, 47.2083)
  line L83 (-2.8867, 47.5725) -> (-1.9913, 50.2327)
  line L84 (-1.9913, 50.2327) -> (-1.5945, 50.2468)
  line L85 (-1.5945, 50.2468) -> (-0.5199, 47.6572)
  line L86 (-0.5199, 47.6572) -> (-0.9989, 47.6401)
  line L87 (-0.9989, 47.6401) -> (-1.7883, 49.6354)
  line L88 (-1.7883, 49.6354) -> (-2.4275, 47.589)
  line L89 (-2.4275, 47.589) -> (-2.8867, 47.5725)
  spline S94 degree 2 poles (-4.4553, 50.1341) (-3.8279, 50.1874) (-3.0786, 49.5423) (-3.0233, 48.8923) knots 0 0 0 1 2 2 2
  spline S95 degree 2 poles (-3.0233, 48.8923) (-2.9691, 48.2536) (-3.5745, 47.4393) (-4.1143, 47.3934) knots 0 0 0 1 2 2 2
  spline S96 degree 2 poles (-4.1143, 47.3934) (-4.3573, 47.3727) (-4.7452, 47.4821) (-4.8964, 47.6201) knots 0 0 0 1 2 2 2
  spline S97 degree 2 poles (-4.8964, 47.6201) (-5.0504, 47.7579) (-5.237, 48.1776) (-5.2636, 48.4913) knots 0 0 0 1 2 2 2
  line L90 (-5.2636, 48.4913) -> (-5.284, 48.7315)
  line L91 (-5.284, 48.7315) -> (-3.4725, 48.8854)
  spline S98 degree 2 poles (-3.4725, 48.8854) (-3.5112, 49.3404) (-4.0101, 49.7848) (-4.417, 49.7502) knots 0 0 0 1 2 2 2
  spline S99 degree 2 poles (-4.417, 49.7502) (-4.5612, 49.738) (-4.8354, 49.6492) (-4.9441, 49.5887) knots 0 0 0 1 2 2 2
  spline S100 degree 2 poles (-4.9441, 49.5887) (-5.058, 49.5221) (-5.2135, 49.4093) (-5.2634, 49.3595) knots 0 0 0 1 2 2 2
  line L92 (-5.2634, 49.3595) -> (-5.2888, 49.3573)
  line L93 (-5.2888, 49.3573) -> (-5.3297, 49.8378)
  spline S101 degree 2 poles (-5.3297, 49.8378) (-5.256, 49.8753) (-5.0319, 49.9855) (-4.9437, 50.0186) knots 0 0 0 1 2 2 2
  spline S102 degree 2 poles (-4.9437, 50.0186) (-4.8196, 50.0661) (-4.6136, 50.1206) (-4.4553, 50.1341) knots 0 0 0 1 2 2 2
  spline S103 degree 2 poles (-4.8259, 48.4317) (-4.8051, 48.2541) (-4.7095, 48.0004) (-4.6314, 47.9188) knots 0 0 0 1 2 2 2
  spline S104 degree 2 poles (-4.6314, 47.9188) (-4.5467, 47.8263) (-4.2976, 47.7422) (-4.1196, 47.7573) knots 0 0 0 1 2 2 2
  spline S105 degree 2 poles (-4.1196, 47.7573) (-3.9444, 47.7722) (-3.7074, 47.8977) (-3.6143, 48.008) knots 0 0 0 1 2 2 2
  spline S106 degree 2 poles (-3.6143, 48.008) (-3.5242, 48.121) (-3.4439, 48.3812) (-3.4439, 48.5491) knots 0 0 0 1 2 2 2
  line L94 (-3.4439, 48.5491) -> (-4.8259, 48.4317)
  line L95 (-6.9438, 47.6228) -> (-6.9213, 47.6257)
  spline S107 degree 2 poles (-6.9213, 47.6257) (-6.8688, 47.6181) (-6.7584, 47.6265) (-6.6824, 47.6362) knots 0 0 0 1 2 2 2
  spline S108 degree 2 poles (-6.6824, 47.6362) (-6.5052, 47.6589) (-6.1761, 47.8583) (-6.038, 48.0304) knots 0 0 0 1 2 2 2
  line L96 (-6.038, 48.0304) -> (-6.2744, 49.8787)
  line L97 (-6.2744, 49.8787) -> (-5.8356, 49.9349)
  line L98 (-5.8356, 49.9349) -> (-5.5023, 47.3297)
  line L99 (-5.5023, 47.3297) -> (-5.9412, 47.2736)
  line L100 (-5.9412, 47.2736) -> (-5.9909, 47.6618)
  spline S109 degree 2 poles (-5.9909, 47.6618) (-6.2026, 47.4174) (-6.5376, 47.1973) (-6.7064, 47.1757) knots 0 0 0 1 2 2 2
  spline S110 degree 2 poles (-6.7064, 47.1757) (-6.774, 47.167) (-6.8422, 47.164) (-6.8855, 47.1671) knots 0 0 0 1 2 2 2
  line L101 (-6.8855, 47.1671) -> (-6.9438, 47.6228)
  spline S111 degree 2 poles (-8.2658, 49.6508) (-8.0056, 49.6944) (-7.5318, 49.6299) (-7.3704, 49.5764) knots 0 0 0 1 2 2 2
  line L102 (-7.3704, 49.5764) -> (-7.2885, 49.0868)
  line L103 (-7.2885, 49.0868) -> (-7.3109, 49.0831)
  spline S112 degree 2 poles (-7.3109, 49.0831) (-7.3743, 49.1185) (-7.5432, 49.1995) (-7.6789, 49.2372) knots 0 0 0 1 2 2 2
  spline S113 degree 2 poles (-7.6789, 49.2372) (-7.7969, 49.2721) (-8.0785, 49.3054) (-8.2212, 49.2816) knots 0 0 0 1 2 2 2
  spline S114 degree 2 poles (-8.2212, 49.2816) (-8.3247, 49.2642) (-8.5545, 49.1769) (-8.6039, 49.1283) knots 0 0 0 1 2 2 2
  spline S115 degree 2 poles (-8.6039, 49.1283) (-8.6761, 49.0616) (-8.7287, 48.9292) (-8.7081, 48.8061) knots 0 0 0 1 2 2 2
  spline S116 degree 2 poles (-8.7081, 48.8061) (-8.6824, 48.6522) (-8.4879, 48.5209) (-8.2636, 48.5038) knots 0 0 0 1 2 2 2
  spline S117 degree 2 poles (-8.2636, 48.5038) (-8.1764, 48.4982) (-7.8985, 48.4872) (-7.7786, 48.4756) knots 0 0 0 1 2 2 2
  spline S118 degree 2 poles (-7.7786, 48.4756) (-7.4676, 48.4386) (-7.1391, 48.1254) (-7.0965, 47.8709) knots 0 0 0 1 2 2 2
  spline S119 degree 2 poles (-7.0965, 47.8709) (-7.0375, 47.5184) (-7.4927, 46.9907) (-7.9291, 46.9177) knots 0 0 0 1 2 2 2
  spline S120 degree 2 poles (-7.9291, 46.9177) (-8.1445, 46.8816) (-8.5987, 46.9149) (-8.7605, 46.9712) knots 0 0 0 1 2 2 2
  line L104 (-8.7605, 46.9712) -> (-8.8387, 47.4384)
  line L105 (-8.8387, 47.4384) -> (-8.8163, 47.4421)
  spline S121 degree 2 poles (-8.8163, 47.4421) (-8.626, 47.3359) (-8.1918, 47.2504) (-7.982, 47.2855) knots 0 0 0 1 2 2 2
  spline S122 degree 2 poles (-7.982, 47.2855) (-7.7666, 47.3216) (-7.5005, 47.5531) (-7.531, 47.7349) knots 0 0 0 1 2 2 2
  spline S123 degree 2 poles (-7.531, 47.7349) (-7.5586, 47.8999) (-7.7615, 48.0299) (-7.9658, 48.0475) knots 0 0 0 1 2 2 2
  spline S124 degree 2 poles (-7.9658, 48.0475) (-8.0651, 48.0567) (-8.3141, 48.0668) (-8.4507, 48.0756) knots 0 0 0 1 2 2 2
  spline S125 degree 2 poles (-8.4507, 48.0756) (-8.7482, 48.1006) (-9.0949, 48.3847) (-9.1431, 48.6729) knots 0 0 0 1 2 2 2
  spline S126 degree 2 poles (-9.1431, 48.6729) (-9.1712, 48.8407) (-9.0893, 49.1593) (-8.9789, 49.2899) knots 0 0 0 1 2 2 2
  spline S127 degree 2 poles (-8.9789, 49.2899) (-8.861, 49.4275) (-8.5315, 49.6063) (-8.2658, 49.6508) knots 0 0 0 1 2 2 2
  line L106 (-10.1124, 49.2446) -> (-9.6786, 49.3317)
  line L107 (-9.6786, 49.3317) -> (-9.1616, 46.7567)
  line L108 (-9.1616, 46.7567) -> (-9.5954, 46.6696)
  line L109 (-9.5954, 46.6696) -> (-10.1124, 49.2446)
  line L110 (-9.5401, 46.2352) -> (-9.0479, 46.334)
  line L111 (-9.0479, 46.334) -> (-8.9574, 45.8835)
  line L112 (-8.9574, 45.8835) -> (-9.4496, 45.7847)
  line L113 (-9.4496, 45.7847) -> (-9.5401, 46.2352)
  spline S128 degree 2 poles (-11.5337, 48.9842) (-11.1825, 49.0646) (-10.6954, 48.7543) (-10.596, 48.3202) knots 0 0 0 1 2 2 2
  line L114 (-10.596, 48.3202) -> (-10.2712, 46.9019)
  line L115 (-10.2712, 46.9019) -> (-9.9809, 46.9683)
  line L116 (-9.9809, 46.9683) -> (-9.8993, 46.6117)
  line L117 (-9.8993, 46.6117) -> (-10.1896, 46.5452)
  line L118 (-10.1896, 46.5452) -> (-10.0212, 45.8098)
  line L119 (-10.0212, 45.8098) -> (-10.4525, 45.711)
  line L120 (-10.4525, 45.711) -> (-10.6209, 46.4465)
  line L121 (-10.6209, 46.4465) -> (-11.4143, 46.2648)
  line L122 (-11.4143, 46.2648) -> (-11.496, 46.6214)
  line L123 (-11.496, 46.6214) -> (-10.7025, 46.8031)
  line L124 (-10.7025, 46.8031) -> (-10.9817, 48.0224)
  spline S129 degree 2 poles (-10.9817, 48.0224) (-11.026, 48.2159) (-11.0886, 48.4256) (-11.1565, 48.5061) knots 0 0 0 1 2 2 2
  spline S130 degree 2 poles (-11.1565, 48.5061) (-11.2136, 48.5774) (-11.4061, 48.6177) (-11.5554, 48.5835) knots 0 0 0 1 2 2 2
  spline S131 degree 2 poles (-11.5554, 48.5835) (-11.6605, 48.5595) (-11.8422, 48.4509) (-11.882, 48.4214) knots 0 0 0 1 2 2 2
  line L125 (-11.882, 48.4214) -> (-11.9069, 48.4157)
  line L126 (-11.9069, 48.4157) -> (-11.9955, 48.8028)
  spline S132 degree 2 poles (-11.9955, 48.8028) (-11.8815, 48.8638) (-11.6415, 48.9595) (-11.5337, 48.9842) knots 0 0 0 1 2 2 2
  line L127 (-13.6196, 45.6726) -> (-13.1974, 49.5107)
  line L128 (-13.1974, 49.5107) -> (-12.7403, 49.6347)
  line L129 (-12.7403, 49.6347) -> (-12.908, 48.4548)
  line L130 (-12.908, 48.4548) -> (-11.3339, 46.2928)
  line L131 (-11.3339, 46.2928) -> (-11.7938, 46.168)
  line L132 (-11.7938, 46.168) -> (-12.9958, 47.8579)
  line L133 (-12.9958, 47.8579) -> (-13.1761, 45.7929)
  line L134 (-13.1761, 45.7929) -> (-13.6196, 45.6726)
  spline S133 degree 2 poles (-17.0296, 47.3658) (-16.672, 47.4944) (-16.1165, 47.5255) (-15.8566, 47.4984) knots 0 0 0 1 2 2 2
  line L135 (-15.8566, 47.4984) -> (-15.6588, 46.9486)
  line L136 (-15.6588, 46.9486) -> (-15.6908, 46.9371)
  spline S134 degree 2 poles (-15.6908, 46.9371) (-15.98, 47.0622) (-16.6077, 47.0895) (-16.8613, 46.9983) knots 0 0 0 1 2 2 2
  spline S135 degree 2 poles (-16.8613, 46.9983) (-17.2242, 46.8677) (-17.4867, 46.4327) (-17.3974, 46.1845) knots 0 0 0 1 2 2 2
  spline S136 degree 2 poles (-17.3974, 46.1845) (-17.3264, 45.987) (-17.0432, 45.8116) (-16.8103, 45.826) knots 0 0 0 1 2 2 2
  spline S137 degree 2 poles (-16.8103, 45.826) (-16.6428, 45.8381) (-16.3681, 45.8706) (-16.1614, 45.8907) knots 0 0 0 1 2 2 2
  spline S138 degree 2 poles (-16.1614, 45.8907) (-15.9742, 45.9068) (-15.6557, 45.8676) (-15.5123, 45.7956) knots 0 0 0 1 2 2 2
  spline S139 degree 2 poles (-15.5123, 45.7956) (-15.3715, 45.7227) (-15.1538, 45.4695) (-15.0846, 45.2773) knots 0 0 0 1 2 2 2
  spline S140 degree 2 poles (-15.0846, 45.2773) (-14.9406, 44.877) (-15.3702, 44.1105) (-15.8533, 43.9367) knots 0 0 0 1 2 2 2
  spline S141 degree 2 poles (-15.8533, 43.9367) (-16.1308, 43.8369) (-16.6613, 43.7696) (-16.9096, 43.7979) knots 0 0 0 1 2 2 2
  line L137 (-16.9096, 43.7979) -> (-17.0977, 44.321)
  line L138 (-17.0977, 44.321) -> (-17.0657, 44.3325)
  spline S142 degree 2 poles (-17.0657, 44.3325) (-16.8564, 44.245) (-16.2885, 44.2082) (-16.019, 44.3052) knots 0 0 0 1 2 2 2
  spline S143 degree 2 poles (-16.019, 44.3052) (-15.7147, 44.4146) (-15.4412, 44.8356) (-15.5247, 45.0677) knots 0 0 0 1 2 2 2
  spline S144 degree 2 poles (-15.5247, 45.0677) (-15.5996, 45.2759) (-15.9104, 45.4444) (-16.1387, 45.4256) knots 0 0 0 1 2 2 2
  spline S145 degree 2 poles (-16.1387, 45.4256) (-16.2909, 45.413) (-16.7285, 45.3641) (-16.8763, 45.3561) knots 0 0 0 1 2 2 2
  spline S146 degree 2 poles (-16.8763, 45.3561) (-17.2527, 45.3383) (-17.7184, 45.644) (-17.8288, 45.9509) knots 0 0 0 1 2 2 2
  spline S147 degree 2 poles (-17.8288, 45.9509) (-17.8989, 46.1457) (-17.8759, 46.576) (-17.7815, 46.7577) knots 0 0 0 1 2 2 2